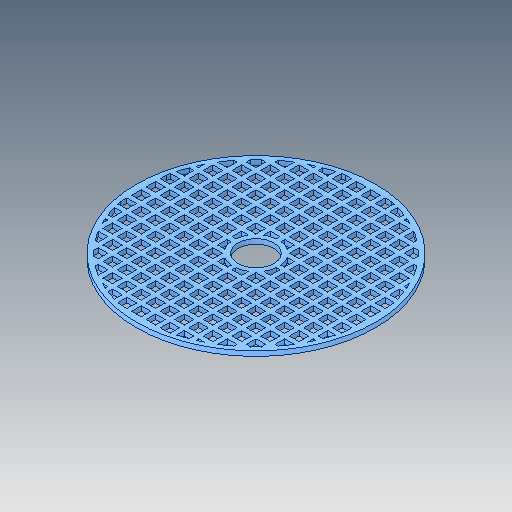
# Autodesk Inventor part: MeshPlate
Saved by Autodesk Inventor 2018 (Build 220112000, 112)
## iProperties
Created: 2017-11-16
Part Number: MeshPlate
Material: Generic
Document SubType Name: Modeling
Designer: Udara Wanasinghe
Density: 1 g/cm^3
Appearance: Default(2)
Mass: 9.1269 g
Surface Area: 163.329 cm^2
Volume: 9.1269 cm^3
Author: Udara Wanasinghe
Autodesk Inventor part; units mm, degrees
ref_plane "YZ Plane" through (0, 0, 0) normal (1, 0, 0) x (0, 1, 0)
ref_plane "XZ Plane" through (0, 0, 0) normal (0, 1, 0) x (-1, 0, 0)
ref_plane "XY Plane" through (0, 0, 0) normal (0, 0, 1) x (1, 0, 0)
sketch "Sketch1" plane through (0, 0, 0) normal (0, 1, 0) x (-1, 0, 0)
  circle A0 centre (0, 0) radius 50
  circle A1 centre (0, 0) radius 48
  dimension "d0" = 100
  dimension "d1" = 96
  constraints: 2 centre point, 2 coincident
  measures "d0" diameter of A0
  measures "d1" diameter of A1
extrude "Extrusion1" add sketch "Sketch1" along normal blind 2
sketch "Sketch3" plane through (0, 0, 0) normal (0, -1, 0) x (1, 0, 0)
  circle A0 centre (0, 0) radius 50
  dimension "d15" = 100
  constraints: 1 centre point, 1 coincident
  measures "d15" diameter of A0
surface extrude "ExtrusionSrf1" sketch "Sketch3" against normal blind 2 shown no curves A0
sketch "Sketch2" plane through (0, 2, 0) normal (0, 1, 0) x (1, 0, 0)
  line L0 (-1, -55.9084) -> (1, -55.9084)
  line L1 (1, -55.9084) -> (1, 55.9084)
  line L2 (1, 55.9084) -> (-1, 55.9084)
  line L3 (-1, 55.9084) -> (-1, -55.9084)
  line L4 (0, -55.9084) -> (0, 55.9084) construction
  point P0 (0, 0)
  point P1 (0, 0)
  dimension "d4" = 2
  constraints: 10 end point, 3 midpoint, 2 parallel, 1 coincident, 1 horizontal, 1 perpendicular
  measures "d4" distance of L2.end L1.end
extrude "Extrusion2" add sketch "Sketch2" against normal blind 2
pattern_linear "Rectangular Pattern1" count 17 spacing 6 along (1, 0, 0) of "Extrusion2" first direction both ways yes
pattern_circular "Circular Pattern1" count 2 over 90 about axis through (0, -10, 0) along (0, 1, 0) of "Extrusion2", "Rectangular Pattern1"
split body "Split1" result one side removed by surface "ExtrusionSrf1" removed pieces at (-51.3028, 0.5, 47.6667) (-51.6412, 0.6667, 6.5) (-51.9628, 0.6667, 0.5) (-51.6412, 0.6667, -6.5) (-35.6667, 1.5, -53.6056) (-6.5, 0.6667, -51.6412) (-0.5, 1.3333, -53.9356) (6.5, 1.3333, -51.6412) (51.3028, 1.5, -36.3333) (53.7748, 1.3333, -6.5) (53.9356, 1.3333, -0.5) (51.6412, 0.6667, 6.5) (48.3333, 1.5, 51.3028) (6.5, 1.3333, 53.7748) (0.5, 1.3333, 53.9356) (-6.5, 1.3333, 51.6412)
sketch "Sketch6" plane through (0, 2, 0) normal (0, 1, 0) x (1, 0, 0)
  circle A0 centre (0, 0) radius 7.5
  dimension "d23" = 15
  constraints: 1 centre point, 1 coincident
  measures "d23" diameter of A0
extrude "Extrusion5" cut sketch "Sketch6" against normal through all
sketch "Sketch7" plane through (0, 2, 0) normal (0, 1, 0) x (1, 0, 0)
  circle A0 centre (0, 0) radius 7.5
  circle A1 centre (0, 0) radius 9.5
  dimension "d26" = 15
  dimension "d27" = 19
  constraints: 2 centre point, 2 coincident
  measures "d26" diameter of A0
  measures "d27" diameter of A1
extrude "Extrusion6" add sketch "Sketch7" against normal blind 2
body "Solid1"
body "Srf1"
